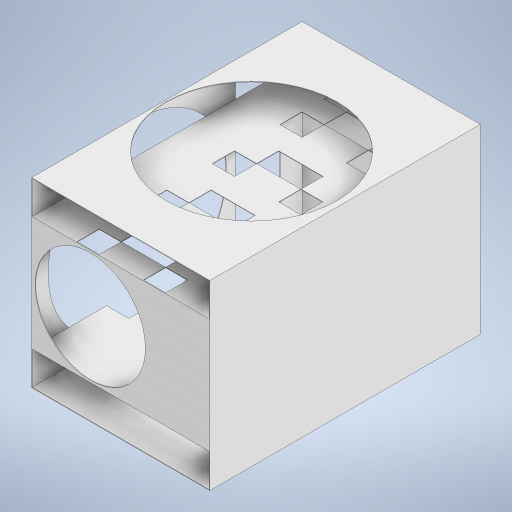
# Autodesk Inventor part: ServerRoom
Saved by Autodesk Inventor 2023.1 (Build 271208000, 208)
## iProperties
Created: 2023-06-06
Part Number: ServerRoom
Material: Gypsum Wall Board
Document SubType Name: Modeling
Designer: rwc6
Density: 1.1 g/cm^3
Appearance: Gypsum Board - Painted White
Author: rwc6
Autodesk Inventor part; units mm, degrees
ref_plane "YZ Plane" through (0, 0, 0) normal (1, 0, 0) x (0, 1, 0)
ref_plane "XZ Plane" through (0, 0, 0) normal (0, 1, 0) x (-1, 0, 0)
sketch "Sketch1" plane through (0, 0, 0) normal (0, 0, 1) x (1, 0, 0)
  line L0 (-2400, -2450) -> (2400, -2450)
  line L1 (2400, -2450) -> (2400, 2450)
  line L2 (2400, 2450) -> (-2400, 2450)
  line L3 (-2400, 2450) -> (-2400, -2450)
  line L4 (-2400, -2450) -> (2400, 2450) construction
  line L5 (2400, -2450) -> (-2400, 2450) construction
  line L6 (-2400, -1550) -> (2400, -1550)
  line L7 (-2400, 1550) -> (2400, 1550)
  line L8 (-2415.875, 2465.875) -> (2415.875, 2465.875)
  line L9 (2415.875, 2465.875) -> (2415.875, -2465.875)
  line L10 (2415.875, -2465.875) -> (-2415.875, -2465.875)
  line L11 (-2415.875, -2465.875) -> (-2415.875, 2465.875)
  line L12 (-2400, -1540) -> (2400, -1540)
  line L13 (-2400, 1560) -> (2400, 1560)
  point P0 (0, 0)
  dimension "d0" = 4800
  dimension "d1" = 4900
  dimension "d2" = 900
  dimension "d3" = 900
  dimension "d4" = 15.875
  dimension "d6" = 10
  dimension "d7" = 10
  constraints: 28 end point, 8 parallel, 4 point on line, 2 midpoint, 2 perpendicular, 1 horizontal, 3 other
  measures "d0" distance of L2.end L1.end
  measures "d1" distance of L1.end L0.end
  measures "d2" distance between parallel lines of L0 L6
  measures "d3" distance between parallel lines of L2 L7
  measures "d4" distance between parallel lines of L2 L8
  measures "d6" distance between parallel lines of L6 L12
  measures "d7" distance between parallel lines of L7 L13
extrude "Extrusion1" add sketch "Sketch1" along normal mid plane 7300 contours L3 L12 L1 L6 | L3 L13 L1 L7 | L8 L9 L10 L11
sketch "Sketch2" plane through (-2415.875, -2465.875, 3650) normal (-1, 0, 0) x (0, 0, 1)
  line L0 (-7300, 4915.875) -> (0, 4915.875) projected
  line L1 (-7300, 4915.875) -> (0, 4915.875) projected
  line L2 (-7300, 15.875) -> (0, 15.875) projected
  line L3 (-7300, 15.875) -> (0, 15.875) projected
  line L4 (-7300, 15.875) -> (0, 15.875) construction
  line L5 (-7300, 15.875) -> (-6100, 15.875) construction
  line L6 (-7300, 15.875) -> (-6100, 15.875) construction
  line L7 (-6100, 15.875) -> (-6100, 2465.875) construction
  line L8 (-7300, 4915.875) -> (0, 4915.875) projected
  line L9 (-6709.6, 15.875) -> (-5490.4, 15.875)
  line L10 (-5490.4, 15.875) -> (-5490.4, 4915.875)
  line L11 (-5490.4, 4915.875) -> (-6709.6, 4915.875)
  line L12 (-6709.6, 4915.875) -> (-6709.6, 15.875)
  line L13 (-6709.6, 15.875) -> (-5490.4, 4915.875) construction
  line L14 (-5490.4, 15.875) -> (-6709.6, 4915.875) construction
  point P0 (-3650, 2465.875)
  point P1 (-6709.6, 4915.875)
  point P2 (-6709.6, 15.875)
  point P3 (-5490.4, 15.875)
  point P4 (-5490.4, 4915.875)
  dimension "d10" = 1200
  dimension "d11" = 0
  dimension "d12" = 2450
  dimension "d13" = 90
  dimension "d14" = 1219.2
  constraints: 18 end point, 2 collinear, 2 horizontal, 2 midpoint, 2 parallel, 2 perpendicular, 1 point on line
  measures "d10" distance of L2.start L5.end
  measures "d11" distance between parallel lines of L5 L6
  measures "d12" distance of L5.end L7.end
  measures "d13" angle of L7 L5
  measures "d14" distance of L11.end L10.end
ref_plane "Work Plane1" through (-2415.875, 0, -2450) normal (0, 1, 0) x (-1, 0, 0)
extrude "Extrusion2" cut sketch "Sketch2" against normal up to surface (15.875 mm away)
sketch "Sketch9" plane through (-2415.875, 0, -2450) normal (0, 1, 0) x (-1, 0, 0)
  line L0 (0, -609.6) -> (0, 609.6) projected
  line L1 (0, 0) -> (-3.2, 0) construction
  line L2 (0, 0) -> (3.2, 0) construction
  point P0 (-2415.875, 2450)
  dimension "d67" = 3.2
  dimension "d68" = 180
  constraints: 4 end point, 2 horizontal, 1 collinear, 1 midpoint
  measures "d67" distance of L1.start L1.end
  measures "d68" angle of L1 L2
sketch "Sketch3" plane through (0, 0, -3650) normal (0, 0, -1) x (-1, 0, 0)
  line L0 (2400, -1540) -> (-2400, -1540) projected
  line L1 (2400, -1540) -> (1800, -1540)
  line L2 (2400, -1540) -> (3000, -1540) construction
  line L3 (-2400, -1540) -> (2400, -1540) projected
  line L4 (-2400, -1540) -> (-1800, -1540)
  line L5 (-2400, -1540) -> (-1800, -1540) construction
  point P0 (0, 0)
  dimension "d17" = 600
  dimension "d18" = 180
  dimension "d19" = 600
  dimension "d20" = 0
  constraints: 8 end point, 4 collinear, 2 horizontal
  measures "d17" distance of L0.start L1.end
  measures "d18" angle of L1 L2
  measures "d19" distance of L0.end L4.end
  measures "d20" distance between parallel lines of L4 L5
sketch "Sketch4" plane through (-2400, 1560, 3650) normal (0, 1, 0) x (1, 0, 0)
  line L0 (4800, 0) -> (4800, 7300) projected
  line L1 (4800, 7300) -> (4800, 0) projected
  line L2 (4800, 0) -> (4800, 7300) construction
  line L3 (4800, 0) -> (3600, 0) construction
  line L4 (0, 0) -> (4800, 0) construction
  line L5 (4800, 0) -> (6000, 0) construction
  line L6 (3600, 0) -> (3000, 0)
  line L7 (3000, 0) -> (3000, 600)
  line L8 (3000, 600) -> (3600, 600)
  line L9 (3600, 600) -> (3600, 0)
  line L10 (3000, 600) -> (2400, 600)
  line L11 (2400, 600) -> (2400, 1200)
  line L12 (2400, 1200) -> (3000, 1200)
  line L13 (3000, 1200) -> (3000, 600)
  point P0 (2400, 3650)
  dimension "d21" = 1200
  dimension "d22" = 180
  dimension "d23" = 600
  dimension "d24" = 600
  dimension "d33" = 600
  dimension "d34" = 600
  constraints: 20 end point, 4 parallel, 3 horizontal, 2 collinear, 2 perpendicular
  measures "d21" distance of L0.start L3.end
  measures "d22" angle of L3 L5
  measures "d23" distance of L7.end L8.end
  measures "d24" distance of L6.end L7.end
  measures "d33" distance of L11.end L12.end
  measures "d34" distance of L10.end L11.end
extrude "Extrusion3" cut sketch "Sketch4" against normal up to surface (10 mm away) contours L6 L7 L8 L9
pattern_linear "Rectangular Pattern1" count 4 spacing 1833.3333 along (0, 0, -1) count 2 spacing 1800 along (-1, 0, 0) of "Extrusion3"
extrude "Extrusion4" cut sketch "Sketch4" against normal up to surface (10 mm away) contours L10 L11 L12 L13
pattern_linear "Rectangular Pattern2" count 2 spacing 600 along (-1, 0, 0) count 4 spacing 1833.3333 along (0, 0, -1) of "Extrusion4"
sketch "Sketch5" plane through (-2400, 1560, -3650) normal (0, 1, 0) x (1, 0, 0)
  line L0 (1800, -600) -> (3000, -600) projected
  line L1 (3000, -600) -> (3600, -600)
  line L2 (3600, -600) -> (3600, 0)
  line L3 (3600, 0) -> (3000, 0)
  line L4 (3000, 0) -> (3000, -600)
  point P0 (2400, -3650)
  dimension "d43" = 600
  dimension "d44" = 600
  constraints: 8 end point, 2 parallel, 1 horizontal, 1 perpendicular
  measures "d43" distance of L3.end L2.end
  measures "d44" distance of L2.end L1.end
extrude "Extrusion5" cut sketch "Sketch5" against normal up to surface (10 mm away)
pattern_linear "Rectangular Pattern3" count 2 spacing 1800 along (-1, 0, 0) of "Extrusion5"
sketch "Sketch6" plane through (-2400, -1540, 3650) normal (0, 1, 0) x (1, 0, 0)
  line L0 (4800, 0) -> (4800, 7300) projected
  line L1 (4800, 7300) -> (4200, 7300)
  line L2 (4200, 7300) -> (4200, 2000)
  line L3 (4200, 2000) -> (4800, 2000)
  line L4 (4800, 2000) -> (4800, 7300)
  point P0 (2400, 3650)
  dimension "d53" = 600
  dimension "d54" = 5300
  constraints: 8 end point, 2 parallel, 1 horizontal, 1 perpendicular
  measures "d53" distance of L3.end L2.end
  measures "d54" distance of L2.end L1.end
extrude "Extrusion6" cut sketch "Sketch6" against normal up to surface (10 mm away)
pattern_linear "Rectangular Pattern4" count 2 spacing 4200 along (-1, 0, 0) of "Extrusion6"
sketch "Sketch7" plane through (0, 0, 3650) normal (0, 0, 1) x (1, 0, 0)
  line L0 (-1200, 1550) -> (-1200, 1560) projected
  line L1 (-1200, 1560) -> (-2400, 1560) projected
  line L2 (-2400, 1560) -> (-2400, 2450) projected
  line L3 (-2400, 2450) -> (2400, 2450) projected
  line L4 (2400, 2450) -> (2400, 1560) projected
  line L5 (2400, 1560) -> (1200, 1560) projected
  line L6 (1200, 1560) -> (1200, 1550) projected
  line L7 (1200, 1550) -> (2400, 1550) projected
  line L8 (2400, 1550) -> (2400, -1540) projected
  line L9 (2400, -1540) -> (-2400, -1540) projected
  line L10 (-2400, -1540) -> (-2400, 1550) projected
  line L11 (-2400, 1550) -> (-1200, 1550) projected
  line L12 (-2415.875, -2465.875) -> (2415.875, -2465.875) projected
  line L13 (2415.875, -2465.875) -> (2415.875, 2465.875) projected
  line L14 (2415.875, 2465.875) -> (-2415.875, 2465.875) projected
  line L15 (-2415.875, 2465.875) -> (-2415.875, -2465.875) projected
  line L16 (2400, -1550) -> (2400, -2450) projected
  line L17 (2400, -2450) -> (-2400, -2450) projected
  line L18 (-2400, -2450) -> (-2400, -1550) projected
  line L19 (-2400, -1550) -> (2400, -1550) projected
  point P0 (0, 0)
extrude "Extrusion7" add sketch "Sketch7" along normal blind 15.875 contours L0 L1 L2 L3 L4 L5 L6 L7 L8 L9 L10 L11 | L15 L14 L13 L12 | L16 L17 L18 L19
sketch "Sketch8" plane through (0, 0, -3650) normal (0, 0, -1) x (-1, 0, 0)
  line L0 (2400, 1550) -> (2400, -2450) projected
  line L1 (2400, -2450) -> (-2400, -2450) projected
  line L2 (-2400, -2450) -> (-2400, 1550) projected
  line L3 (-2400, 1550) -> (-1200, 1550) projected
  line L4 (-1200, 1550) -> (-1200, 1560) projected
  line L5 (-1200, 1560) -> (-2400, 1560) projected
  line L6 (-2400, 1560) -> (-2400, 2450) projected
  line L7 (-2400, 2450) -> (2400, 2450) projected
  line L8 (2400, 2450) -> (2400, 1560) projected
  line L9 (2400, 1560) -> (1200, 1560) projected
  line L10 (1200, 1560) -> (1200, 1550) projected
  line L11 (1200, 1550) -> (2400, 1550) projected
  line L12 (-2415.875, -2465.875) -> (2415.875, -2465.875) projected
  line L13 (2415.875, -2465.875) -> (2415.875, 2465.875) projected
  line L14 (2415.875, 2465.875) -> (-2415.875, 2465.875) projected
  line L15 (-2415.875, 2465.875) -> (-2415.875, -2465.875) projected
  point P0 (0, 0)
extrude "Extrusion8" add sketch "Sketch8" along normal blind 15.875 contours L0 L1 L2 L3 L4 L5 L6 L7 L8 L9 L10 L11 | L15 L14 L13 L12
sketch "Sketch10" plane through (-2415.875, -2465.875, 3665.875) normal (-1, 0, 0) x (0, 0, 1)
  circle A0 centre (-2847.1158, 2465.875) radius 2419.0506
  point P0 (-3665.875, 2465.875)
  constraints: 1 centre point
extrude "Extrusion9" cut sketch "Sketch10" against normal blind 15.875
sketch "Sketch11" plane through (-2415.875, 2465.875, 3665.875) normal (0, 1, 0) x (1, 0, 0)
  circle A0 centre (2359.9202, 3600.5944) radius 2321.7481
  point P0 (2415.875, 3665.875)
  constraints: 1 centre point
extrude "Extrusion10" cut sketch "Sketch11" against normal blind 15.875
sketch "Sketch13" plane through (0, 0, 3665.875) normal (0, 0, 1) x (1, 0, 0)
  line L0 (-2400, 1560) -> (-1200, 1560) projected
  line L1 (-1200, 1560) -> (-2400, 1560) projected
  line L2 (-1200, 1560) -> (-600, 1560) projected
  line L3 (-600, 1560) -> (600, 1560) projected
  line L4 (600, 1560) -> (1200, 1560) projected
  line L5 (2400, 1560) -> (1200, 1560) projected
  line L6 (1200, 1560) -> (2400, 1560) projected
  line L7 (1200, 1560) -> (600, 1560) projected
  line L8 (600, 1560) -> (1200, 1560) projected
  line L9 (1200, 1560) -> (600, 1560) projected
  line L10 (600, 1560) -> (-600, 1560) projected
  line L11 (-600, 1560) -> (-1200, 1560) projected
  line L12 (-1200, 1560) -> (-600, 1560) projected
  line L13 (-600, 1560) -> (-1200, 1560) projected
  line L14 (-600, 1560) -> (-1200, 1560) projected
  line L15 (-1200, 1560) -> (-600, 1560) projected
  line L16 (-600, 1560) -> (600, 1560) projected
  line L17 (600, 1560) -> (1200, 1560) projected
  line L18 (1200, 1560) -> (600, 1560) projected
  line L19 (600, 1560) -> (-600, 1560) projected
  line L20 (-600, 1560) -> (-1200, 1560) projected
  line L21 (-1200, 1560) -> (-600, 1560) projected
  line L22 (-600, 1560) -> (600, 1560) projected
  line L23 (600, 1560) -> (1200, 1560) projected
  line L24 (1200, 1560) -> (600, 1560) projected
  line L25 (600, 1560) -> (-600, 1560) projected
  line L26 (600, 1560) -> (-600, 1560) projected
  line L27 (600, 1560) -> (-600, 1560) projected
  line L28 (-2400, 1560) -> (-2400, 1560) projected
  line L29 (-2400, 1560) -> (-2400, 2450) projected
  line L30 (-2400, 1560) -> (-2400, 2450) projected
  line L31 (2265.7933, 2450) -> (-2377.7029, 2450) projected
  line L32 (-2400, 2450) -> (2400, 2450) projected
  line L33 (-2415.875, 2450) -> (-2400, 2450) projected
  line L34 (-2415.875, 2450) -> (-2400, 2450) projected
  line L35 (2400, 2450) -> (-2400, 2450) projected
  line L36 (-2400, -1550) -> (2400, -1550) projected
  line L37 (2400, -1550) -> (2400, -2450) projected
  line L38 (2400, -2450) -> (-2400, -2450) projected
  line L39 (-2400, -2450) -> (-2400, -1550) projected
  line L40 (2400, 2450) -> (2400, 1560) projected
  line L41 (2400, 1560) -> (2400, 2450) projected
  circle A0 centre (-826.4052, 0) radius 1495.9981
  point P0 (0, 0)
  constraints: 1 centre point
extrude "Extrusion12" cut sketch "Sketch13" against normal blind 15.875
equation "\"d4\" = out_w_thick"
equation "\"d6\" = flr_clng_thick"
equation "\"d7\" = flr_clng_thick"
equation "\"d12\" = 0.5 * win_h"
equation "\"d14\" = win_w"
equation "\"d67\" = 0.5 * win_d"
equation "\"d63\" = out_w_thick"
equation "\"d65\" = out_w_thick"
equation "\"d69\" = out_w_thick"
equation "\"d71\" = out_w_thick"
equation "\"d75\" = out_w_thick"
equation "\"out_w_thick\" = 15.875"
equation "\"flr_clng_thick\" = 10"
equation "\"win_h\" = 4900"
equation "\"win_w\" = 1219.2"
equation "\"win_d\" = 6.4"
